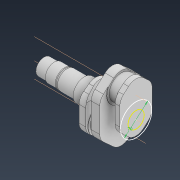
# Autodesk Inventor part: Korbowód poprawiony
Saved by Autodesk Inventor 2022 (Build 260153000, 153)
## iProperties
Created: 2023-04-16
Part Number: Korbowód poprawiony
Material: Generic
Document SubType Name: Modeling
Designer: wikto
Density: 1 g/cm^3
Appearance: Default
Author: wikto
Autodesk Inventor part; units mm, degrees
ref_plane "YZ Plane" through (0, 0, 0) normal (1, 0, 0) x (0, 1, 0)
ref_plane "XZ Plane" through (0, 0, 0) normal (0, 1, 0) x (-1, 0, 0)
ref_plane "XY Plane" through (0, 0, 0) normal (0, 0, 1) x (1, 0, 0)
sketch "Sketch1" plane through (0, 0, 0) normal (0, 0, 1) x (1, 0, 0)
  line L0 (0, 0) -> (115.5, 0)
  line L1 (0, 0) -> (0, 18)
  line L2 (0, 18) -> (23, 18)
  line L3 (23, 18) -> (23, 20)
  line L4 (23, 20) -> (46, 20)
  line L5 (46, 20) -> (46, 21)
  line L6 (46, 21) -> (48, 21)
  arc A0 (48, 21) -> (51, 21) centre (49.5, 21) ccw
  line L7 (51, 21) -> (90, 21)
  line L8 (90, 21) -> (90, 25)
  line L9 (115.5, 32.5) -> (115.5, 0)
  line L10 (90, 25) -> (114.5, 25)
  line L11 (114.5, 25) -> (114.5, 32.5)
  line L12 (114.5, 32.5) -> (115.5, 32.5)
  dimension "d1" = 23
  dimension "d2" = 23
  dimension "d3" = 44
  dimension "d4" = 36
  dimension "d6" = 40
  dimension "d7" = 42
  dimension "d9" = 25.5
  dimension "d10" = 2
  dimension "d11" = 1.5
  dimension "d13" = 65
  dimension "d14" = 50
  dimension "d15" = 1
  constraints: 26 end point, 8 perpendicular, 3 horizontal, 3 horizontal alignment, 2 point on circle, 1 centre point, 1 vertical
  measures "d1" distance between parallel lines of L3 L1
  measures "d2" distance between parallel lines of L5 L3
  measures "d3" distance between parallel lines of L8 L5
  measures "d4" diameter of L2 L0
  measures "d6" diameter of L4 L0
  measures "d7" diameter of L7 L0
  measures "d9" distance between parallel lines of L8 L9
  measures "d10" distance of L5.end L6.end
  measures "d11" radius of A0
  measures "d13" diameter of L12 L0
  measures "d14" diameter of L10 L0
  measures "d15" distance between parallel lines of L9 L11
revolve "Revolution1" add sketch "Sketch1" angle 360 about axis through (0, 0, 0) along (1, 0, 0)
sketch "Sketch3" plane through (115.5, 0, 0) normal (1, 0, 0) x (0, 0, -1)
  arc A0 (14.7825, 31.9413) -> (-14.7825, 31.9413) centre (0, 11.78) ccw
  line L0 (-14.7825, 31.9413) -> (-26.7825, 23.1427)
  line L1 (14.7825, 31.9413) -> (26.7825, 23.1427)
  arc A1 (-26.7825, 23.1427) -> (-37, 2.9815) centre (-12, 2.9815) ccw
  arc A2 (37, 2.9815) -> (26.7825, 23.1427) centre (12, 2.9815) ccw
  line L2 (-37, 2.9815) -> (-37, -33.4185)
  line L3 (37, -33.4185) -> (37, 2.9815)
  arc A3 (-37, -33.4185) -> (-26.7825, -53.5798) centre (-12, -33.4185) ccw
  arc A4 (26.7825, -53.5798) -> (37, -33.4185) centre (12, -33.4185) ccw
  circle A5 centre (0, 0) radius 32.5 construction
  line L4 (-33.5015, 15.7363) -> (-5.6983, 36.1219) construction
  line L5 (-26.7825, -53.5798) -> (-14.7825, -62.3784)
  line L6 (26.7825, -53.5798) -> (14.7825, -62.3784)
  arc A6 (-14.7825, -62.3784) -> (14.7825, -62.3784) centre (0, -42.2171) ccw
  dimension "d17" = 25
  dimension "d18" = 74
  dimension "d19" = 36.4
  dimension "d21" = 14.88
  dimension "d24" = 2
  dimension "d50" = 14.88
  constraints: 14 end point, 14 point on circle, 10 tangent, 6 centre point, 5 equal radius, 3 equal length, 3 horizontal alignment, 2 vertical, 2 vertical alignment, 1 parallel
  measures "d17" radius of A0
  measures "d18" distance between parallel lines of L3 L2
  measures "d19" distance of L2.start L2.end
  measures "d21" distance of L1.end L1.start
  measures "d24" distance between parallel lines of L0 L4
  measures "d50" distance of L6.start L6.end
extrude "Extrusion6" add sketch "Sketch3" along normal blind 14.76
sketch "Sketch10" plane through (115.5, -33.4185, 37) normal (0, 0, 1) x (1, 0, 0)
  line L0 (-1, 0.9185) -> (0, 0.9185) projected
  line L1 (0, -9.3815) -> (6.106, -33.7985)
  line L2 (6.106, -33.7985) -> (0, -33.7985)
  line L3 (0, -20.1613) -> (0, 0) projected
  line L4 (0, -33.7985) -> (0, -9.3815)
  line L5 (0, -20.1613) -> (0, -28.9598) projected
  line L6 (0, -33.7985) -> (14.76, -33.7985) construction
  line L7 (0, 70.1985) -> (14.76, 70.1985) projected
  line L8 (7.38, 70.1985) -> (7.38, -33.7985) construction
  line L9 (0, 0) -> (0, 36.4) projected
  line L10 (0, 18.2) -> (14.76, 18.2) construction
  line L11 (14.76, -9.3815) -> (8.654, -33.7985) construction
  line L12 (8.654, -33.7985) -> (14.76, -33.7985) construction
  line L13 (14.76, -33.7985) -> (14.76, -9.3815) construction
  line L14 (14.76, 18.2) -> (0, 18.2) construction
  line L15 (8.654, 70.1985) -> (14.76, 70.1985)
  line L16 (14.76, 70.1985) -> (14.76, 45.7815)
  line L17 (14.76, 45.7815) -> (8.654, 70.1985)
  point P0 (-115.5, 33.4185)
  point P1 (0, -24.5606)
  point P2 (3.053, -33.7985)
  point P3 (0, -9.3815)
  point P4 (8.654, 70.1985)
  dimension "d53" = 10.3
  dimension "d54" = 165.96
  constraints: 24 end point, 8 symmetric about line, 5 midpoint, 2 perpendicular, 2 point on line, 1 horizontal
  measures "d53" distance of L1.start L0.end
  measures "d54" angle of L1 L3
extrude "Extrusion7" cut sketch "Sketch10" against normal through all
sketch "Sketch11" plane through (130.26, 0, 0) normal (1, 0, 0) x (0, 0, -1)
  line L0 (-26.7825, -53.5798) -> (-14.7825, -62.3784) projected
  arc A0 (26.7825, -53.5798) -> (-26.7825, -53.5798) centre (0, -35.1693) ccw
  line L1 (14.7825, -62.3784) -> (26.7825, -53.5798) projected
  arc A1 (-14.7825, -62.3784) -> (14.7825, -62.3784) centre (0, -42.2171) ccw projected
  dimension "d58" = 32.5
  constraints: 2 point on circle, 1 centre point
  measures "d58" radius of A0
extrude "Extrusion8" add sketch "Sketch11" along normal blind 1
sketch "Sketch12" plane through (131.26, 0, 0) normal (1, 0, 0) x (0, 0, -1)
  arc A0 (26.7825, -53.5798) -> (-26.7825, -53.5798) centre (0, -35.1693) ccw projected
  circle A1 centre (0, -35.1693) radius 27.5
  point P0 (0, 0)
  dimension "d61" = 55
  constraints: 1 centre point, 1 coincident
  measures "d61" diameter of A1
extrude "Extrusion9" add sketch "Sketch12" along normal blind 21
sketch "Sketch13" plane through (152.26, -35.1693, 0) normal (1, 0, 0) x (0, 0, -1)
  circle A0 centre (0, 0) radius 32.5
  circle A1 centre (0, 0) radius 27.5 projected
  point P0 (0, 35.1693)
  dimension "d64" = 65
  constraints: 1 centre point, 1 coincident
  measures "d64" diameter of A0
extrude "Extrusion10" add sketch "Sketch13" along normal blind 1 contours A0 | A1
sketch "Sketch14" plane through (153.26, -35.1693, 0) normal (1, 0, 0) x (0, 0, -1)
  line L0 (-47.5, 13.3355) -> (-47.5, 68.7355)
  line L1 (-39.2847, 87.2632) -> (-16.7847, 107.6465)
  line L2 (39.2847, 87.2632) -> (16.7847, 107.6465)
  line L3 (47.5, 68.7355) -> (47.5, 13.3355)
  line L4 (-39.2847, -5.1921) -> (-16.7847, -25.5755)
  line L5 (39.2847, -5.1921) -> (16.7847, -25.5755)
  arc A0 (-47.5, 13.3355) -> (-39.2847, -5.1921) centre (-22.5, 13.3355) ccw
  arc A1 (-16.7847, -25.5755) -> (16.7847, -25.5755) centre (0, -7.0478) ccw
  arc A2 (39.2847, -5.1921) -> (47.5, 13.3355) centre (22.5, 13.3355) ccw
  arc A3 (47.5, 68.7355) -> (39.2847, 87.2632) centre (22.5, 68.7355) ccw
  arc A4 (-39.2847, 87.2632) -> (-47.5, 68.7355) centre (-22.5, 68.7355) ccw
  arc A5 (16.7847, 107.6465) -> (-16.7847, 107.6465) centre (0, 89.1188) ccw
  arc A6 (-14.7825, -27.2091) -> (14.7825, -27.2091) centre (0, -7.0478) ccw projected
  point P0 (0, 35.1693)
  dimension "d67" = 25
  dimension "d68" = 55.4
  dimension "d71" = 30.36
  dimension "d72" = 95
  constraints: 13 tangent, 12 end point, 12 point on circle, 6 centre point, 5 equal radius, 4 equal length, 3 horizontal alignment, 2 vertical
  measures "d67" radius of A5
  measures "d68" distance of L3.start L3.end
  measures "d71" distance of L2.start L2.end
  measures "d72" distance between parallel lines of L3 L0
extrude "Extrusion11" add sketch "Sketch14" along normal blind 18.91
sketch "Sketch15" plane through (172.17, -35.1693, 0) normal (1, 0, 0) x (0, 0, -1)
  arc A0 (16.7847, 107.6465) -> (-16.7847, 107.6465) centre (0, 89.1188) ccw projected
  line L0 (-16.7847, 107.6465) -> (-39.2847, 87.2632) projected
  line L1 (39.2847, 87.2632) -> (16.7847, 107.6465) projected
  arc A1 (-29.2427, 96.3605) -> (29.2427, 96.3605) centre (0, 82.179) ccw
  point P0 (0, 35.1693)
  dimension "d76" = 32.5
  dimension "d77" = 13.55
  constraints: 2 point on circle, 2 point on line, 1 centre point, 1 vertical alignment
  measures "d76" radius of A1
  measures "d77" distance of A1.start L0.end
extrude "Extrusion12" add sketch "Sketch15" along normal blind 1
sketch "Sketch16" plane through (173.17, -35.1693, 0) normal (1, 0, 0) x (0, 0, -1)
  line L0 (-16.7847, 107.6465) -> (-29.2427, 96.3605) projected
  arc A0 (-29.2427, 96.3605) -> (29.2427, 96.3605) centre (0, 82.179) ccw projected
  line L1 (29.2427, 96.3605) -> (16.7847, 107.6465) projected
  arc A1 (16.7847, 107.6465) -> (-16.7847, 107.6465) centre (0, 89.1188) ccw projected
  circle A2 centre (0, 82.179) radius 27.5
  point P0 (0, 35.1693)
  dimension "d80" = 55
  constraints: 1 centre point, 1 coincident
  measures "d80" diameter of A2
extrude "Extrusion13" add sketch "Sketch16" along normal blind 21 contours A2
sketch "Sketch17" plane through (153.26, -35.1693, 0) normal (1, 0, 0) x (0, 0, -1)
  line L0 (-16.7847, -25.5755) -> (-29.1479, -14.3753) projected
  arc A0 (-29.1479, -14.3753) -> (29.1479, -14.3753) centre (0, 0) ccw projected
  line L1 (29.1479, -14.3753) -> (16.7847, -25.5755) projected
  arc A1 (-16.7847, -25.5755) -> (16.7847, -25.5755) centre (0, -7.0478) ccw projected
  point P0 (0, 35.1693)
extrude "Extrusion14" cut sketch "Sketch17" against normal blind 2
sketch "Sketch18" plane through (194.17, 47.0097, 0) normal (1, 0, 0) x (0, 0, -1)
  arc A0 (-29.2427, 14.1815) -> (29.2427, 14.1815) centre (0, 0) ccw projected
  circle A1 centre (0, 0) radius 32.5
  point P0 (0, -47.0097)
  point P1 (29.2427, 14.1815)
  point P2 (-29.2427, 14.1815)
  dimension "d85" = 65
  constraints: 1 centre point, 1 coincident
  measures "d85" diameter of A1
extrude "Extrusion15" add sketch "Sketch18" along normal blind 1
sketch "Sketch19" plane through (195.17, 47.0097, 0) normal (1, 0, 0) x (0, 0, -1)
  arc A0 (16.7847, 25.4675) -> (-16.7847, 25.4675) centre (0, 6.9399) ccw projected
  arc A1 (16.7847, 25.4675) -> (-16.7847, 25.4675) centre (0, 6.9399) ccw projected
  line L0 (-16.7847, 25.4675) -> (-27.9013, 15.3967)
  line L1 (16.7847, 25.4675) -> (27.9013, 15.3967)
  arc A2 (-27.9013, 15.3967) -> (-36.1166, -3.1309) centre (-11.1166, -3.1309) ccw
  arc A3 (36.1166, -3.1309) -> (27.9013, 15.3967) centre (11.1166, -3.1309) ccw
  line L2 (36.1166, -3.1309) -> (36.1166, -43.5309)
  line L3 (-36.1166, -3.1309) -> (-36.1166, -43.5309)
  arc A4 (27.9013, -62.0586) -> (36.1166, -43.5309) centre (11.1166, -43.5309) ccw
  arc A5 (-36.1166, -43.5309) -> (-27.9013, -62.0586) centre (-11.1166, -43.5309) ccw
  line L4 (27.9013, -62.0586) -> (16.7847, -72.1294)
  line L5 (-27.9013, -62.0586) -> (-16.7847, -72.1294)
  arc A6 (-16.7847, -72.1294) -> (16.7847, -72.1294) centre (0, -53.6018) ccw
  point P0 (0, -47.0097)
  dimension "d88" = 15
  dimension "d89" = 25
  dimension "d90" = 40.4
  constraints: 12 end point, 11 tangent, 10 point on circle, 5 centre point, 4 equal radius, 3 equal length, 3 horizontal alignment, 2 vertical
  measures "d88" distance of L0.start L0.end
  measures "d89" radius of A3
  measures "d90" distance of L3.start L3.end
extrude "Extrusion16" add sketch "Sketch19" along normal blind 10.43
sketch "Sketch20" plane through (195.17, 47.0097, 0) normal (1, 0, 0) x (0, 0, -1)
  arc A0 (29.3356, 13.9883) -> (27.9013, 15.3967) centre (11.1166, -3.1309) ccw projected
  arc A1 (29.3356, 13.9883) -> (-29.3356, 13.9883) centre (0, 0) ccw projected
  arc A2 (-27.9013, 15.3967) -> (-29.3356, 13.9883) centre (-11.1166, -3.1309) ccw projected
  line L0 (-27.9013, 15.3967) -> (-16.7847, 25.4675) projected
  arc A3 (16.7847, 25.4675) -> (-16.7847, 25.4675) centre (0, 6.9399) ccw projected
  line L1 (16.7847, 25.4675) -> (27.9013, 15.3967) projected
  point P0 (0, -47.0097)
extrude "Extrusion17" cut sketch "Sketch20" against normal blind 10.43
sketch "Sketch21" plane through (205.6, 47.0097, 0) normal (1, 0, 0) x (0, 0, -1)
  circle A0 centre (0, -47.0097) radius 35
  circle A1 centre (0, -47.0097) radius 18 projected
  dimension "d95" = 70
  constraints: 2 coincident, 1 centre point
  measures "d95" diameter of A0
body "Solid1"
